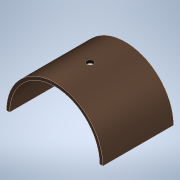
# Autodesk Inventor part: Под шатун
Saved by Autodesk Inventor 2021 (Build 250183000, 183)
## iProperties
Created: 2020-12-10
Part Number: Под шатун
Material: Бронза, литейная
Document SubType Name: Modeling
Designer: Тимоха
Mass: 1108.04 g
Surface Area: 534.85 cm^2
Volume: 124.92 cm^3
Density: 8.87 g/cm^3
Appearance: Бронза - сатинированная
Author: Тимоха
Autodesk Inventor part; units mm, degrees
ref_plane "YZ Plane" through (0, 0, 0) normal (1, 0, 0) x (0, 1, 0)
ref_plane "XZ Plane" through (0, 0, 0) normal (0, 1, 0) x (-1, 0, 0)
ref_plane "XY Plane" through (0, 0, 0) normal (0, 0, 1) x (1, 0, 0)
sketch "Эскиз1" plane through (0, 0, 0) normal (0, 0, 1) x (1, 0, 0)
  circle A0 centre (0, 0) radius 75
  circle A1 centre (0, 0) radius 70
  line L0 (-75, 0) -> (75, 0)
  point P0 (70, 0)
  point P1 (-70, 0)
  dimension "d0" = 150
  dimension "d1" = 140
  constraints: 2 centre point, 2 coincident, 2 end point, 2 point on circle
  measures "d0" diameter of A0
  measures "d1" diameter of A1
extrude "Выдавливание1" add sketch "Эскиз1" along normal blind 110 contours L0 A1 A0 picked at (0, 71.5073)
sketch "Эскиз2" plane through (0, 0, 0) normal (0, 1, 0) x (-1, 0, 0)
  line L0 (-75, 0) -> (75, 0) projected
  line L1 (75, 0) -> (75, 110) projected
  line L2 (-75, 110) -> (75, 110) projected
  line L3 (-75, 0) -> (-75, 110) projected
  circle A0 centre (0, 55) radius 5
  point P0 (0, 0)
  dimension "d4" = 10
  constraints: 1 centre point
  measures "d4" diameter of A0
extrude "Выдавливание2" cut sketch "Эскиз2" along normal blind 110 contours A0
